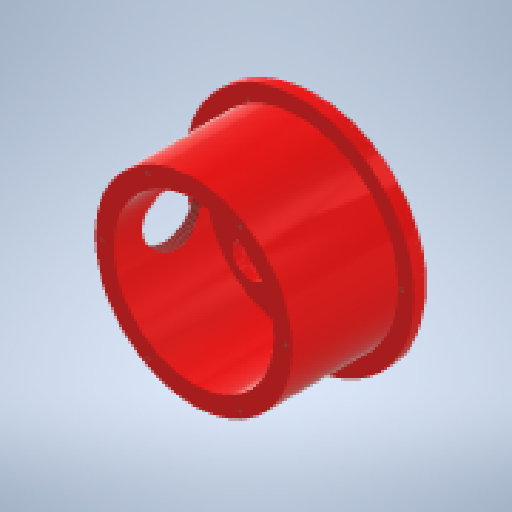
# Autodesk Inventor part: 021
Saved by Autodesk Inventor 2023 (Build 270158000, 158)
## iProperties
Created: 2021-11-06
Part Number: 021
Material: Stainless Steel, 440C
Document SubType Name: Modeling
Designer: vinicius.miguel
Density: 7.75 g/cm^3
Appearance: Smooth - Red
Mass: 1833.41 g
Surface Area: 585.078 cm^2
Volume: 236.569 cm^3
Author: vinicius.miguel
Autodesk Inventor part; units mm, degrees
ref_plane "XZ Plane" through (0, 0, 0) normal (0, 1, 0) x (-1, 0, 0)
ref_plane "XY Plane" through (0, 0, 0) normal (0, 0, 1) x (1, 0, 0)
sketch "Sketch1" plane through (0, 0, 0) normal (1, 0, 0) x (0, 1, 0)
  line L0 (0, 0) -> (0, 16.4674) construction
  line L1 (-57, -4.6) -> (-57, 0)
  line L2 (-57, 0) -> (-60, 0)
  line L3 (-60, 0) -> (-60, 5.4)
  line L4 (-60, 5.4) -> (-44.45, 5.4)
  line L5 (-44.45, 5.4) -> (-44.45, 2)
  line L6 (-44.45, 2) -> (-41.5, 2)
  line L7 (-41.5, -4.6) -> (-57, -4.6)
  line L8 (-41.5, -4.6) -> (-41.5, 2)
  line L9 (-51.5, 5.4) -> (-51.5, 60.4)
  line L10 (-51.5, 60.4) -> (-41.5, 60.4)
  line L11 (-41.5, 60.4) -> (-41.5, 2)
  line L12 (-45, 60.4) -> (-45, 59.2)
  line L13 (-45, 59.2) -> (-43, 59.2)
  line L14 (-43, 59.2) -> (-43, 60.4)
  line L15 (-41.5, 11.4) -> (-14, 11.4)
  line L16 (-14, 11.4) -> (-14, 7.4)
  line L17 (-14, 7.4) -> (-41.5, 7.4)
  point P0 (-47.5615, 5.4)
  dimension "d2" = 4.6
  dimension "d3" = 10
  dimension "d8" = 88.9
  dimension "d9" = 120
  dimension "d20" = 114
  dimension "d40" = 2
  dimension "d44" = 83
  dimension "d45" = 65
  dimension "d46" = 10
  dimension "d68" = 86
  dimension "d69" = 2
  dimension "d70" = 1.2
  dimension "d81" = 4
  dimension "d82" = 12
  dimension "d83" = 28
  constraints: 36 end point, 12 perpendicular, 5 point on line, 4 vertical, 1 horizontal, 1 horizontal alignment
  measures "d2" distance of L1.start L1.end
  measures "d3" distance between parallel lines of L4 L7
  measures "d8" diameter of L5 L0
  measures "d9" diameter of L3 L0
  measures "d20" diameter of L1 L0
  measures "d40" distance between parallel lines of L2 L6
  measures "d44" diameter of L11 L0
  measures "d45" distance between parallel lines of L7 L10
  measures "d46" distance of L9.end L10.end
  measures "d68" diameter of L14 L0
  measures "d69" distance of L12.end L13.end
  measures "d70" distance of L13.end L14.end
  measures "d81" distance of L15.end L16.end
  measures "d82" distance between parallel lines of L17 L7
  measures "d83" diameter of L16 L0
revolve "Revolution1" add sketch "Sketch1" angle 360 about axis through (0, 0, 0) along (0, 0, 1)
chamfer "Chamfer4" distance 1 angle 45 1 edges at (0, 57, -4.6)
sketch "Sketch2" plane through (0, 0, -4.6) normal (0, 0, -1) x (-1, 0, 0)
  point P0 (0, 0)
  point P1 (-53, 0)
  dimension "d26" = 53
  constraints: 1 horizontal alignment
  measures "d26" distance of point (0, 0) point (-53, 0)
hole "Hole1" at (53, 0, -4.6) direction (0, 0, 1) diameter 2.459 end through all counterbore diameter 4 counterbore depth 4.6 thread size "M3x0.5" class "6H" standard "ANSI Metric M Profile"
pattern_circular "Circular Pattern1" count 3 over 360 about axis through (0, 0, 2.7) along (0, 0, 1) of "Hole1"
chamfer "Chamfer5" distance 3 angle 45 1 edges at (0, 41.5, -4.6)
sketch "Sketch3" plane through (0, 0, 60.4) normal (0, 0, 1) x (1, 0, 0)
  circle A0 centre (0, 0) radius 51.5 projected
  circle A1 centre (0, 0) radius 41.5 projected
  circle A2 centre (0, 0) radius 51.5 projected
  point P0 (48, 0)
  dimension "d65" = 48
  constraints: 1 horizontal alignment
  measures "d65" distance of point (48, 0) point (0, 0)
hole "Hole2" at (48, 0, 60.4) direction (0, 0, -1) diameter 2.459 depth 8.8 tip angle 118 thread size "M3x0.5" class "6H" standard "ISO Metric profile"
pattern_circular "Circular Pattern2" count 6 over 360 about axis through (0, 0, 32.9) along (0, 0, 1) of "Hole2"
ref_plane "Work Plane1" through (-51.5, 0, 32.9) normal (1, 0, 0) x (0, 1, 0)
sketch "Sketch4" plane through (-51.5, 0, 32.9) normal (1, 0, 0) x (0, 1, 0)
  circle A0 centre (0, -2.5) radius 15
  line L0 (60, -27.5) -> (-60, -27.5) projected
  point P0 (0, -32.9)
  dimension "d57" = 30
  dimension "d58" = 25
  constraints: 1 centre point, 1 vertical alignment
  measures "d57" diameter of A0
  measures "d58" distance from line of A0.centre L0
extrude "Extrusion1" cut sketch "Sketch4" along normal blind 15
chamfer "Chamfer6" distance 0.25 angle 45 4 edges at (0, 51.5, 60.4) (0, 41.5, 60.4) (0, 60, 5.4) (0, 60, 0)
sketch "Sketch5" plane through (-51.5, 0, 32.9) normal (1, 0, 0) x (0, 1, 0)
  line L0 (51.5, -27.5) -> (-51.5, -27.5) projected
  line L1 (51.5, 27.25) -> (-51.5, 27.25) projected
  line L2 (-51.5, -27.5) -> (-51.5, 27.25) projected
  line L3 (51.5, -27.5) -> (51.5, 27.25) projected
  line L4 (51.5, -27.5) -> (51.5, 27.25) projected
  line L5 (51.5, 18.5) -> (-51.5, 18.5)
  line L6 (-51.5, -27.5) -> (-51.5, 27.25) projected
  line L7 (51.5, -27.5) -> (51.5, 27.25) projected
  line L8 (51.5, -23.5) -> (-51.5, -23.5)
  line L9 (-51.5, -27.5) -> (-51.5, 27.25) projected
  point P0 (0, -32.9)
  point P1 (51.5, 18.5)
  point P2 (-51.5, 18.5)
  dimension "d72" = 6
  dimension "d73" = 6
  constraints: 4 end point, 2 perpendicular, 2 point on line, 2 vertical alignment, 4 other
  measures "d72" distance from line of L5 point (0, 12.5)
  measures "d73" distance from line of L8 point (0, -17.5)
extrude "Extrusion2" cut sketch "Sketch5" along normal blind 6 contours L8 L2 L5 L3
sketch "Sketch6" plane through (-45.5, 0, 32.9) normal (-1, 0, 0) x (0, 0, 1)
  circle A0 centre (-2.5, 0) radius 15 projected
  point P0 (-32.9, 0)
  constraints: 1 coincident
hole "Hole3" at (-45.5, 0, 30.4) direction (1, 0, 0) diameter 30.3762 depth 25 tip angle 118 thread size "M32x1.5" class "6H" standard "ISO Metric profile"
sketch "Sketch7" plane through (0, 0, 7.4) normal (0, 0, -1) x (-1, 0, 0)
  circle A0 centre (27.75, 0) radius 9
  circle A1 centre (0, 0) radius 41.5 projected
  circle A2 centre (0, 0) radius 14 projected
  circle A3 centre (0, 0) radius 41.5 projected
  line L0 (41.5, 0) -> (14, 0) construction
  dimension "d84" = 18
  constraints: 3 horizontal alignment, 2 end point, 1 centre point, 1 coincident, 1 horizontal, 1 midpoint, 2 other
  measures "d84" diameter of A0
extrude "Extrusion3" cut sketch "Sketch7" against normal blind 10 contours A0
pattern_circular "Circular Pattern3" count 8 over 360 about axis through (0, 0, 9.4) along (0, 0, 1) of "Extrusion3"
equation "\"d73\" = d72"
body "Solid1"
